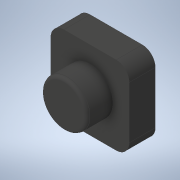
# Autodesk Inventor part: Button
Saved by Autodesk Inventor 2020.1 (Build 241239000, 239)
## iProperties
Created: 2019-10-05
Part Number: Button
Material: PET Plastic
Document SubType Name: Modeling
Designer: Josiah
Density: 1.541 g/cm^3
Appearance: Generic
Author: Josiah
Autodesk Inventor part; units mm, degrees
ref_plane "YZ Plane" through (0, 0, 0) normal (1, 0, 0) x (0, 1, 0)
ref_plane "XZ Plane" through (0, 0, 0) normal (0, 1, 0) x (-1, 0, 0)
ref_plane "XY Plane" through (0, 0, 0) normal (0, 0, 1) x (1, 0, 0)
sketch "Sketch1" plane through (0, 0, 0) normal (0, 0, 1) x (1, 0, 0)
  line L0 (6, -6) -> (-6, -6)
  line L1 (-6, -6) -> (-6, 6)
  line L2 (-6, 6) -> (6, 6)
  line L3 (6, 6) -> (6, -6)
  point P0 (0, 0)
  point P1 (0, 0)
  dimension "d0" = 12
  dimension "d1" = 12
  dimension "d2" = 6
  dimension "d3" = 6
  constraints: 8 end point, 2 parallel, 1 coincident, 1 horizontal, 1 perpendicular, 2 other
  measures "d0" distance of L0.start L0.end
  measures "d1" distance of L0.end L1.end
  measures "d2" distance from line of point (0, 0) L0
  measures "d3" distance from line of point (0, 0) L1
extrude "Extrusion1" add sketch "Sketch1" along normal blind 4
fillet "Fillet1" radius 2 4 edges at (-6, 6, 2) (-6, -6, 2) (6, 6, 2) (6, -6, 2)
sketch "Sketch2" plane through (0, 0, 4) normal (0, 0, 1) x (1, 0, 0)
  circle A0 centre (0, 0) radius 3.5
  dimension "d7" = 7
  constraints: 2 coincident, 1 centre point, 2 other
  measures "d7" diameter of A0
extrude "Extrusion2" add sketch "Sketch2" along normal blind 4
fillet "Fillet2" radius 0.5 1 edges at (-3.5, 0, 8)
body "Solid1"
